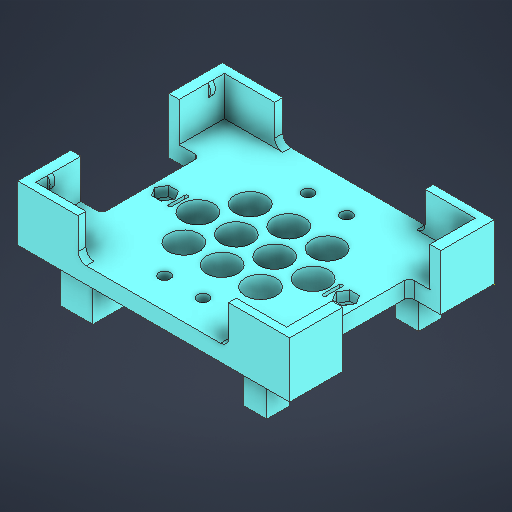
# Autodesk Inventor part: PILLARSCELLCASE18650
Saved by Autodesk Inventor 2026.2 (Build 302298000, 298)
## iProperties
Created: 2024-11-21
Part Number: PILLARSCELLCASE18650
Material: Generic
Document SubType Name: Modeling
Designer: cbast
Density: 1 g/cm^3
Appearance: Default
Mass: 190.937 g
Surface Area: 666.623 cm^2
Volume: 190.937 cm^3
Author: cbast
## iProperties of the stored document BatteryCasev1_3DPrint.ipt
Created: 2025-01-30
Part Number: BatteryCasev1_3DPrint
Material: Generic
Document SubType Name: Modeling
Designer: cbast
Density: 1 g/cm^3
Appearance: Default
Author: cbast
Autodesk Inventor part; units mm, degrees
ref_plane "YZ Plane" through (0, 0, 0) normal (1, 0, 0) x (0, 1, 0)
ref_plane "XZ Plane" through (0, 0, 0) normal (0, 1, 0) x (-1, 0, 0)
ref_plane "XY Plane" through (0, 0, 0) normal (0, 0, 1) x (1, 0, 0)
sketch "Sketch1" plane through (0, 0, 0) normal (0, 1, 0) x (-1, 0, 0)
  circle A0 centre (0, 0) radius 9.5
  circle A1 centre (23.5, 0) radius 9.5
  circle A2 centre (-23.5, 0) radius 9.5
  circle A3 centre (47, 0) radius 9.5
  line L0 (0, 0) -> (-32.9562, 0) construction
  line L1 (-32.9562, 0) -> (61.076, 0) construction
  circle A4 centre (0, 0) radius 14 construction
  circle A5 centre (-23.5, 0) radius 14 construction
  circle A6 centre (47, 0) radius 14 construction
  circle A7 centre (23.5, 0) radius 14 construction
  circle A8 centre (47, 0) radius 15 construction
  circle A9 centre (-23.5, 0) radius 15 construction
  circle A10 centre (0, 0) radius 15 construction
  circle A11 centre (23.5, 0) radius 15 construction
  line L2 (37.5, 0) -> (33, 0) construction
  circle A12 centre (35.25, -20.3516) radius 9.5
  circle A13 centre (35.25, -20.3516) radius 14 construction
  circle A14 centre (35.25, -20.3516) radius 15 construction
  line L3 (14, 0) -> (9.5, 0) construction
  line L4 (-9.5, 0) -> (-14, 0) construction
  line L5 (35.25, -20.3516) -> (-11.75, -20.3516) construction
  circle A15 centre (11.75, -20.3516) radius 9.5
  circle A16 centre (-11.75, -20.3516) radius 9.5
  circle A17 centre (11.75, -20.3516) radius 14 construction
  circle A18 centre (11.75, -20.3516) radius 15 construction
  circle A19 centre (-11.75, -20.3516) radius 14 construction
  circle A20 centre (-11.75, -20.3516) radius 15 construction
  circle A21 centre (35.25, 20.3516) radius 9.5
  circle A22 centre (35.25, 20.3516) radius 14 construction
  circle A23 centre (35.25, 20.3516) radius 15 construction
  line L6 (35.25, 20.3516) -> (-11.75, 20.3516) construction
  circle A24 centre (11.75, 20.3516) radius 9.5
  circle A25 centre (-11.75, 20.3516) radius 9.5
  circle A26 centre (11.75, 20.3516) radius 14 construction
  circle A27 centre (11.75, 20.3516) radius 15 construction
  circle A28 centre (-11.75, 20.3516) radius 14 construction
  circle A29 centre (-11.75, 20.3516) radius 15 construction
  arc A30 (49.1998, -14.8378) -> (49.1998, 14.8378) centre (47, 0) ccw
  arc A31 (49.1998, 14.8378) -> (23.5, 29.6756) centre (35.25, 20.3516) ccw
  arc A32 (23.5, 29.6756) -> (0, 29.6756) centre (11.75, 20.3516) ccw
  arc A33 (0, 29.6756) -> (-25.6998, 14.8378) centre (-11.75, 20.3516) ccw
  arc A34 (-25.6998, 14.8378) -> (-25.6998, -14.8378) centre (-23.5, 0) ccw
  arc A35 (-25.6998, -14.8378) -> (0, -29.6756) centre (-11.75, -20.3516) ccw
  arc A36 (0, -29.6756) -> (23.5, -29.6756) centre (11.75, -20.3516) ccw
  arc A37 (23.5, -29.6756) -> (49.1998, -14.8378) centre (35.25, -20.3516) ccw
  point P0 (46.8931, -14.9996)
  point P1 (46.8931, 14.9996)
  point P2 (-23.3931, 14.9996)
  point P3 (-23.3931, -14.9996)
  dimension "d145" = 28
  dimension "d149" = 28
  dimension "d0" = 19
  dimension "d2" = 19
  dimension "d4" = 19
  dimension "d53" = 19
  dimension "d144" = 28
  dimension "d150" = 28
  dimension "d154" = 30
  dimension "d158" = 30
  dimension "d162" = 30
  dimension "d163" = 30
  dimension "d291" = 19
  dimension "d292" = 28
  dimension "d293" = 30
  dimension "d294" = 19
  dimension "d295" = 19
  dimension "d296" = 28
  dimension "d297" = 30
  dimension "d298" = 28
  dimension "d299" = 30
  constraints: 40 point on circle, 36 centre point, 32 coincident, 12 end point, 10 vertical alignment, 9 equal radius, 4 tangent, 2 horizontal alignment, 1 horizontal, 1 midpoint, 1 parallel, 1 point on line, 17 other
  measures "d0" diameter of A0
  measures "d2" diameter of A1
  measures "d4" diameter of A2
  measures "d53" diameter of A3
  measures "d144" diameter of A4
  measures "d150" diameter of A7
  measures "d154" diameter of A8
  measures "d158" diameter of A9
  measures "d162" diameter of A10
  measures "d163" diameter of A11
  measures "d291" diameter of A12
  measures "d292" diameter of A13
  measures "d293" diameter of A14
  measures "d294" diameter of A15
  measures "d295" diameter of A16
  measures "d296" diameter of A17
  measures "d297" diameter of A18
  measures "d298" diameter of A19
  measures "d299" diameter of A20
extrude "Extrusion1" add sketch "Sketch1" along normal blind 15
sketch "Sketch26" plane through (0, 15, 0) normal (0, 1, 0) x (1, 0, 0)
  arc A0 (-49.1998, -14.8378) -> (-23.5, -29.6756) centre (-35.25, -20.3516) ccw projected
  arc A1 (-23.5, -29.6756) -> (0, -29.6756) centre (-11.75, -20.3516) ccw projected
  arc A2 (0, -29.6756) -> (25.6998, -14.8378) centre (11.75, -20.3516) ccw projected
  arc A3 (25.6998, -14.8378) -> (25.6998, 14.8378) centre (23.5, 0) ccw projected
  arc A4 (25.6998, 14.8378) -> (0, 29.6756) centre (11.75, 20.3516) ccw projected
  arc A5 (0, 29.6756) -> (-23.5, 29.6756) centre (-11.75, 20.3516) ccw projected
  arc A6 (-23.5, 29.6756) -> (-49.1998, 14.8378) centre (-35.25, 20.3516) ccw projected
  arc A7 (-49.1998, 14.8378) -> (-49.1998, -14.8378) centre (-47, 0) ccw projected
  circle A8 centre (0, 0) radius 9.5 projected
  circle A9 centre (-23.5, 0) radius 9.5 projected
  circle A10 centre (11.75, -20.3516) radius 9.5 projected
  circle A11 centre (-11.75, -20.3516) radius 9.5 projected
  circle A12 centre (-35.25, -20.3516) radius 9.5 projected
  circle A13 centre (11.75, 20.3516) radius 9.5 projected
  circle A14 centre (-11.75, 20.3516) radius 9.5 projected
  circle A15 centre (-35.25, 20.3516) radius 9.5 projected
  circle A16 centre (-47, 0) radius 9.5 projected
  circle A17 centre (23.5, 0) radius 9.5 projected
  line L0 (-88.45, 57.7) -> (64.95, 57.7)
  line L1 (64.95, 57.7) -> (64.95, -57.7)
  line L2 (64.95, -57.7) -> (-88.45, -57.7)
  line L3 (-88.45, -57.7) -> (-88.45, 57.7)
  line L4 (-88.45, 57.7) -> (64.95, -57.7) construction
  line L5 (64.95, 57.7) -> (-88.45, -57.7) construction
  line L6 (-88.45, 0) -> (-62, 0) construction
  line L7 (38.5, 0) -> (64.95, 0) construction
  point P0 (-11.75, 0)
  dimension "d300" = 153.4
  dimension "d301" = 115.4
  constraints: 16 end point, 4 midpoint, 3 equal length, 2 horizontal, 2 point on circle, 1 collinear, 1 perpendicular
  measures "d300" distance of L1.end L2.end
  measures "d301" distance of L0.end L1.end
extrude "Extrusion24" add sketch "Sketch26" against normal blind 10 contours L0 L1 L2 L3
sketch "Sketch28" plane through (0, 15, 0) normal (0, 1, 0) x (1, 0, 0)
  line L0 (-88.45, -57.7) -> (64.95, -57.7) projected
  line L1 (64.95, -57.7) -> (64.95, 57.7) projected
  line L2 (64.95, 57.7) -> (-88.45, 57.7) projected
  line L3 (-88.45, 57.7) -> (-88.45, -57.7) projected
  circle A0 centre (0, 0) radius 9.5 projected
  circle A1 centre (-23.5, 0) radius 9.5 projected
  circle A2 centre (11.75, -20.3516) radius 9.5 projected
  circle A3 centre (-11.75, -20.3516) radius 9.5 projected
  circle A4 centre (-35.25, -20.3516) radius 9.5 projected
  circle A5 centre (11.75, 20.3516) radius 9.5 projected
  circle A6 centre (-11.75, 20.3516) radius 9.5 projected
  circle A7 centre (-35.25, 20.3516) radius 9.5 projected
  circle A8 centre (-47, 0) radius 9.5 projected
  circle A9 centre (23.5, 0) radius 9.5 projected
  line L4 (64.95, 57.7) -> (64.95, -57.7) projected
  line L5 (-88.0641, -57.4308) -> (64.95, -57.4308)
  line L6 (64.95, -57.4308) -> (64.95, 57.7)
  line L7 (64.95, 57.7) -> (-88.0641, 57.7)
  line L8 (-88.0641, 57.7) -> (-88.0641, -57.4308)
  line L9 (-88.0641, -57.4308) -> (64.95, 57.7) construction
  line L10 (64.95, -57.4308) -> (-88.0641, 57.7) construction
  line L11 (-94.7093, -62.4308) -> (71.5952, -62.4308)
  line L12 (71.5952, -62.4308) -> (71.5952, 62.7)
  line L13 (71.5952, 62.7) -> (-94.7093, 62.7)
  line L14 (-94.7093, 62.7) -> (-94.7093, -62.4308)
  line L15 (-94.7093, -62.4308) -> (71.5952, 62.7) construction
  line L16 (71.5952, -62.4308) -> (-94.7093, 62.7) construction
  point P0 (-11.5571, 0.1346)
  point P1 (-11.5571, 0.1346)
  dimension "d306" = 5
  constraints: 24 end point, 5 midpoint, 4 parallel, 2 horizontal, 2 perpendicular, 1 point on line
  measures "d306" distance between parallel lines of L13 L2
extrude "Extrusion25" add sketch "Sketch28" along normal blind 24 and the other way blind 10 contours L14 L13 L12 L11
sketch "Sketch29" plane through (-94.7093, 39, 62.4308) normal (0, 0, 1) x (1, 0, 0)
  line L0 (6.2593, -24) -> (159.6593, -24) projected
  line L1 (41.9593, -24) -> (123.9593, -24)
  line L2 (166.3046, 0) -> (0, 0) projected
  line L3 (128.9593, -24) -> (36.9593, -24)
  line L4 (36.9593, -19) -> (36.9593, 0)
  line L5 (36.9593, 0) -> (128.9593, 0)
  line L6 (128.9593, 0) -> (128.9593, -19)
  arc A0 (36.9593, -19) -> (41.9593, -24) centre (41.9593, -19) ccw
  arc A1 (123.9593, -24) -> (128.9593, -19) centre (123.9593, -19) ccw
  point P0 (94.7093, -39)
  point P1 (82.9593, -24)
  point P2 (42.9593, -24)
  point P3 (128.9593, 0)
  dimension "d311" = 86
  dimension "d312" = 5
  constraints: 10 end point, 6 point on line, 4 point on circle, 4 tangent, 2 centre point, 2 midpoint, 2 parallel, 1 equal radius, 1 horizontal, 1 perpendicular
  measures "d311" distance of point (42.959, -24) L3.start
  measures "d312" radius of A0
extrude "Extrusion26" cut sketch "Sketch29" against normal through all
sketch "Sketch30" plane through (0, 39, 0) normal (0, 1, 0) x (1, 0, 0)
  circle A0 centre (-47, 0) radius 9.5 projected
  circle A1 centre (0, 0) radius 9.5 projected
  circle A2 centre (-23.5, 0) radius 9.5 projected
  circle A3 centre (11.75, -20.3516) radius 9.5 projected
  circle A4 centre (-11.75, -20.3516) radius 9.5 projected
  circle A5 centre (-35.25, -20.3516) radius 9.5 projected
  circle A6 centre (11.75, 20.3516) radius 9.5 projected
  circle A7 centre (-11.75, 20.3516) radius 9.5 projected
  circle A8 centre (-35.25, 20.3516) radius 9.5 projected
  circle A9 centre (23.5, 0) radius 9.5 projected
  line L0 (29.25, -57.7) -> (64.95, -57.7) projected
  line L1 (64.95, -57.7) -> (64.95, 57.7) projected
  line L2 (64.95, 57.7) -> (29.25, 57.7) projected
  line L3 (29.25, 57.7) -> (29.25, 62.7) projected
  line L4 (-52.75, 62.7) -> (29.25, 62.7) projected
  line L5 (-52.75, 57.7) -> (-52.75, 62.7) projected
  line L6 (-52.75, 57.7) -> (-88.45, 57.7) projected
  line L7 (-88.45, 57.7) -> (-88.45, -57.7) projected
  line L8 (-88.45, -57.7) -> (-52.75, -57.7) projected
  line L9 (-52.75, -62.4308) -> (-52.75, -57.7) projected
  line L10 (29.25, -62.4308) -> (-52.75, -62.4308) projected
  line L11 (29.25, -62.4308) -> (29.25, -57.7) projected
  line L12 (34.25, -57.7) -> (34.25, -62.4308) projected
  line L13 (34.25, -62.4308) -> (71.5952, -62.4308) projected
  line L14 (71.5952, -62.4308) -> (71.5952, 62.7) projected
  line L15 (71.5952, 62.7) -> (34.25, 62.7) projected
  line L16 (34.25, 62.7) -> (34.25, 57.7) projected
  line L17 (34.25, 57.7) -> (64.95, 57.7) projected
  line L18 (64.95, 57.7) -> (64.95, -57.7) projected
  line L19 (64.95, -57.7) -> (34.25, -57.7) projected
  line L20 (-88.45, -57.7) -> (-88.45, 57.7) projected
  line L21 (-57.75, -62.4308) -> (-57.75, -57.7) projected
  line L22 (-57.75, -57.7) -> (-88.45, -57.7) projected
  line L23 (-88.45, -57.7) -> (-88.45, 57.7) projected
  line L24 (-88.45, 57.7) -> (-57.75, 57.7) projected
  line L25 (-57.75, 57.7) -> (-57.75, 62.7) projected
  line L26 (-57.75, 62.7) -> (-94.7093, 62.7) projected
  line L27 (-94.7093, 62.7) -> (-94.7093, -62.4308) projected
  line L28 (-94.7093, -62.4308) -> (-57.75, -62.4308) projected
  line L29 (-88.45, -30) -> (-88.45, 30)
  line L30 (-94.7093, -62.4308) -> (-94.7093, 62.7) projected
  line L31 (-75.7093, 27) -> (-75.7093, -27)
  arc A10 (-75.7093, 27) -> (-78.7093, 30) centre (-78.7093, 27) ccw
  arc A11 (-78.7093, -30) -> (-75.7093, -27) centre (-78.7093, -27) ccw
  line L32 (-94.7093, 0) -> (-47, 0) construction
  line L33 (-47, 0) -> (-94.7093, 0) construction
  line L34 (-78.7093, 30) -> (-114.521, 30)
  line L35 (-114.521, 30) -> (-114.521, -30)
  line L36 (-114.521, -30) -> (-78.7093, -30)
  point P0 (-88.45, 0)
  dimension "d317" = 3
  constraints: 14 end point, 4 point on circle, 3 perpendicular, 2 centre point, 2 midpoint, 2 tangent, 1 collinear, 1 equal radius, 1 horizontal
  measures "d317" radius of A10
extrude "Extrusion27" cut sketch "Sketch30" against normal through all contours L36 L27 L34 L7 | L7 L34 A10 L31 A11 L36 | L36 L35 L34 L27
ref_plane "Work Plane9" through (-11.75, 15, -57.7) normal (-1, 0, 0) x (0, 0, 1)
sketch "Sketch31" plane through (0, 15, 0) normal (0, 1, 0) x (1, 0, 0)
  line L0 (-64.06, 5.3) -> (-61, 0)
  line L1 (-61, 0) -> (-64.06, -5.3)
  line L2 (-64.06, -5.3) -> (-70.1799, -5.3)
  line L3 (-70.1799, -5.3) -> (-73.2398, 0)
  line L4 (-73.2398, 0) -> (-70.1799, 5.3)
  line L5 (-70.1799, 5.3) -> (-64.06, 5.3)
  line L6 (-88.45, 57.7) -> (-57.75, 57.7) projected
  circle A0 centre (-47, 0) radius 9.5 projected
  line L7 (-57.75, -57.7) -> (-88.45, -57.7) projected
  line L8 (-75.7093, -27) -> (-75.7093, 27) construction
  line L9 (-75.7093, 0) -> (-47, 0) construction
  point P0 (0, 0)
  point P1 (-67.1199, 0)
  dimension "d323" = 14
  dimension "d332" = 10.6
  constraints: 14 end point, 2 parallel, 1 midpoint, 1 perpendicular, 1 point on line, 13 other
  measures "d323" distance of L9.end L0.end
  measures "d332" distance between parallel lines of L2 L5
extrude "Extrusion28" cut sketch "Sketch31" against normal blind 6 contours L0 L1 L2 L3 L4 L5
sketch "Sketch32" plane through (0, 9, 0) normal (0, 1, 0) x (1, 0, 0)
  line L0 (-73.2398, 0) -> (-70.1799, 5.3) projected
  line L1 (-70.1799, -5.3) -> (-73.2398, 0) projected
  line L2 (-64.06, -5.3) -> (-70.1799, -5.3) projected
  line L3 (-61, 0) -> (-64.06, -5.3) projected
  line L4 (-64.06, 5.3) -> (-61, 0) projected
  line L5 (-70.1799, 5.3) -> (-64.06, 5.3) projected
  circle A0 centre (-67.1199, 0) radius 3.25
  line L6 (-63.8699, 0) -> (-61, 0) construction
  line L7 (-70.3699, 0) -> (-73.2398, 0) construction
  point P0 (0, 0)
  dimension "d329" = 6.5
  constraints: 4 end point, 2 collinear, 2 point on circle, 1 centre point, 1 horizontal, 1 point on line
  measures "d329" diameter of A0
extrude "Extrusion29" cut sketch "Sketch32" against normal through all contours A0
sketch "Sketch33" plane through (0, 15, 0) normal (0, 1, 0) x (1, 0, 0)
  line L0 (-70.1799, -5.3) -> (-73.2398, 0) projected
  line L1 (-73.2398, 0) -> (-70.1799, 5.3) projected
  line L2 (-70.1799, 5.3) -> (-64.06, 5.3) projected
  line L3 (-64.06, 5.3) -> (-61, 0) projected
  line L4 (-61, 0) -> (-64.06, -5.3) projected
  line L5 (-64.06, -5.3) -> (-70.1799, -5.3) projected
  circle A0 centre (23.5, 0) radius 9.5 projected
  circle A1 centre (-35.25, 20.3516) radius 9.5 projected
  circle A2 centre (-11.75, 20.3516) radius 9.5 projected
  circle A3 centre (11.75, 20.3516) radius 9.5 projected
  circle A4 centre (-35.25, -20.3516) radius 9.5 projected
  circle A5 centre (-11.75, -20.3516) radius 9.5 projected
  circle A6 centre (11.75, -20.3516) radius 9.5 projected
  circle A7 centre (-23.5, 0) radius 9.5 projected
  circle A8 centre (0, 0) radius 9.5 projected
  circle A9 centre (-47, 0) radius 9.5 projected
  line L6 (64.95, -57.7) -> (64.95, 57.7) projected
  line L7 (64.95, 57.7) -> (29.25, 57.7) projected
  line L8 (29.25, 57.7) -> (29.25, 62.7) projected
  line L9 (-52.75, 62.7) -> (29.25, 62.7) projected
  line L10 (-52.75, 57.7) -> (-52.75, 62.7) projected
  line L11 (-52.75, 57.7) -> (-88.45, 57.7) projected
  line L12 (-88.45, 57.7) -> (-88.45, 30) projected
  line L13 (-88.45, -57.7) -> (-52.75, -57.7) projected
  line L14 (-52.75, -62.4308) -> (-52.75, -57.7) projected
  line L15 (29.25, -62.4308) -> (-52.75, -62.4308) projected
  line L16 (29.25, -62.4308) -> (29.25, -57.7) projected
  line L17 (29.25, -57.7) -> (64.95, -57.7) projected
  line L18 (-59, 6) -> (-59, -6) construction
  line L19 (-60, 5) -> (-60, -5)
  line L20 (-58, -5) -> (-58, 5)
  arc A10 (-58, 5) -> (-60, 5) centre (-59, 5) ccw
  arc A11 (-60, -5) -> (-58, -5) centre (-59, -5) ccw
  line L21 (-47, 0) -> (-75.7093, 0) construction
  line L22 (-88.45, 30) -> (-78.7093, 30) projected
  arc A12 (-75.7093, 27) -> (-78.7093, 30) centre (-78.7093, 27) ccw projected
  line L23 (-75.7093, 27) -> (-75.7093, -27) projected
  arc A13 (-78.7093, -30) -> (-75.7093, -27) centre (-78.7093, -27) ccw projected
  line L24 (-78.7093, -30) -> (-88.45, -30) projected
  line L25 (-88.45, -30) -> (-88.45, -57.7) projected
  point P0 (-59, 0)
  dimension "d333" = 12
  dimension "d334" = 2
  dimension "d335" = 11
  constraints: 10 end point, 6 point on circle, 4 tangent, 3 point on line, 2 centre point, 1 midpoint, 1 parallel, 1 vertical
  measures "d333" distance of L18.start L18.end
  measures "d334" diameter of A11
  measures "d335" distance from line of L20 L21.start
extrude "Extrusion30" cut sketch "Sketch33" against normal through all contours A10 L20 A11 L19
mirror "Mirror9" about plane through (-11.75, 15, -57.7) normal (-1, 0, 0) of "Extrusion28", "Extrusion29", "Extrusion30"
ref_plane "Work Plane10" through (-94.7093, 5, -0.1346) normal (0, 0, 1) x (1, 0, 0)
ref_plane "Work Plane11" through (64.95, 15, -47.7) normal (0, 0, 1) x (1, 0, 0)
sketch "Sketch34" plane through (64.95, 15, -47.7) normal (0, 0, 1) x (1, 0, 0)
  line L0 (0, 24) -> (0, 0) projected
  line L1 (0, 0) -> (0, 16) construction
  line L2 (0, 0) -> (0, 24) construction
  line L3 (0, 16) -> (0, 24)
  arc A0 (0, 24) -> (0, 16) centre (0, 20) ccw
  arc A1 (0, 24) -> (0, 16) centre (4.4721, 20) ccw
  point P0 (-64.95, -15)
  dimension "d339" = 16
  dimension "d340" = 8
  dimension "d342" = 6
  constraints: 4 end point, 4 point on circle, 2 centre point, 2 point on line
  measures "d339" distance of L0.end L1.end
  measures "d340" distance of L1.end L3.end
  measures "d342" radius of A1
extrude "Extrusion31" add sketch "Sketch34" against normal blind 3 contours L0 A1
mirror "Mirror10" about plane through (-11.75, 15, -57.7) normal (-1, 0, 0) of "Extrusion31"
mirror "Mirror11" about plane through (-94.7093, 5, -0.1346) normal (0, 0, 1) of "Extrusion31", "Mirror10"
sketch "Sketch35" plane through (0, 5, 0) normal (0, -1, 0) x (1, 0, 0)
  line L0 (-94.7093, -62.7) -> (71.5952, -62.7) projected
  point P0 (0, 0)
sketch "Sketch36" plane through (0, 15, 0) normal (0, 1, 0) x (1, 0, 0)
  line L0 (-88.45, 30) -> (-78.7093, 30) construction
  line L1 (-78.7093, -30) -> (-88.45, -30) construction
  line L2 (-75.7093, 27) -> (-75.7093, -27) construction
  line L3 (64.95, 47.7) -> (64.95, -47.4308) construction
  line L4 (71.5952, 62.7) -> (71.5952, -62.4308) construction
  line L5 (64.95, 20.5623) -> (52.209, 20.5623) construction
  line L6 (-75.7093, -2.0148) -> (-75.7093, -47.4308) construction
  line L7 (52.24, 27) -> (52.24, -27)
  line L8 (55.24, -30) -> (114.3089, -30)
  line L9 (114.3089, -30) -> (114.3089, 30)
  line L10 (114.3089, 30) -> (55.24, 30)
  arc A0 (55.24, 30) -> (52.24, 27) centre (55.24, 27) ccw
  arc A1 (52.24, -27) -> (55.24, -30) centre (55.24, -27) ccw
  point P0 (0, 0)
  dimension "d347" = 12.741
  dimension "d348" = 3
  constraints: 12 end point, 4 point on circle, 4 tangent, 3 perpendicular, 3 point on line, 2 centre point, 1 equal radius, 1 horizontal, 1 vertical
  measures "d347" distance of L5.start L5.end
  measures "d348" radius of A0
extrude "Extrusion32" cut sketch "Sketch36" along normal through all both and the other way through all
sketch "Sketch37" plane through (0, 5, 0) normal (0, -1, 0) x (1, 0, 0)
  line L0 (-72.2093, 38.9308) -> (-57.2093, 38.9308)
  line L1 (-57.2093, 38.9308) -> (-57.2093, 53.9308)
  line L2 (-57.2093, 53.9308) -> (-72.2093, 53.9308)
  line L3 (-72.2093, 53.9308) -> (-72.2093, 38.9308)
  line L4 (-72.2093, 38.9308) -> (-57.2093, 53.9308) construction
  line L5 (-57.2093, 38.9308) -> (-72.2093, 53.9308) construction
  line L6 (-74.7093, 36.4308) -> (-54.7093, 36.4308)
  line L7 (-54.7093, 36.4308) -> (-54.7093, 56.4308)
  line L8 (-54.7093, 56.4308) -> (-74.7093, 56.4308)
  line L9 (-74.7093, 56.4308) -> (-74.7093, 36.4308)
  line L10 (-74.7093, 36.4308) -> (-54.7093, 56.4308) construction
  line L11 (-54.7093, 36.4308) -> (-74.7093, 56.4308) construction
  line L12 (-94.7093, 62.4308) -> (-94.7093, 30) projected
  line L13 (71.5952, 62.4308) -> (-94.7093, 62.4308) projected
  line L14 (34.5952, 39.4308) -> (48.5952, 39.4308)
  line L15 (48.5952, 39.4308) -> (48.5952, 53.4308)
  line L16 (48.5952, 53.4308) -> (34.5952, 53.4308)
  line L17 (34.5952, 53.4308) -> (34.5952, 39.4308)
  line L18 (34.5952, 39.4308) -> (48.5952, 53.4308) construction
  line L19 (48.5952, 39.4308) -> (34.5952, 53.4308) construction
  line L20 (71.5952, 30) -> (71.5952, 62.4308) projected
  line L21 (-75.7093, -27) -> (-75.7093, 27) construction
  line L22 (-75.7093, 0) -> (52.24, 0) construction
  line L23 (52.24, -27) -> (52.24, 27) construction
  line L24 (-72.2093, -38.9308) -> (-57.2093, -38.9308)
  line L25 (-57.2093, -38.9308) -> (-57.2093, -53.9308)
  line L26 (-57.2093, -53.9308) -> (-72.2093, -53.9308)
  line L27 (-72.2093, -53.9308) -> (-72.2093, -38.9308)
  line L28 (-72.2093, -38.9308) -> (-57.2093, -53.9308) construction
  line L29 (-57.2093, -38.9308) -> (-72.2093, -53.9308) construction
  line L30 (-74.7093, -36.4308) -> (-54.7093, -36.4308)
  line L31 (-54.7093, -36.4308) -> (-54.7093, -56.4308)
  line L32 (-54.7093, -56.4308) -> (-74.7093, -56.4308)
  line L33 (-74.7093, -56.4308) -> (-74.7093, -36.4308)
  line L34 (-74.7093, -36.4308) -> (-54.7093, -56.4308) construction
  line L35 (-54.7093, -36.4308) -> (-74.7093, -56.4308) construction
  line L36 (34.5952, -39.4308) -> (48.5952, -39.4308)
  line L37 (48.5952, -39.4308) -> (48.5952, -53.4308)
  line L38 (48.5952, -53.4308) -> (34.5952, -53.4308)
  line L39 (34.5952, -53.4308) -> (34.5952, -39.4308)
  line L40 (34.5952, -39.4308) -> (48.5952, -53.4308) construction
  line L41 (48.5952, -39.4308) -> (34.5952, -53.4308) construction
  point P0 (0, 0)
  point P1 (-64.7093, 46.4308)
  point P2 (41.5952, 46.4308)
  point P3 (-64.7093, -46.4308)
  point P4 (41.5952, -46.4308)
  dimension "d351" = 15
  dimension "d352" = 20
  dimension "d355" = 16
  dimension "d356" = 30
  dimension "d357" = 14
  dimension "d358" = 14
  dimension "d359" = 16
  dimension "d360" = 30
  constraints: 74 end point, 14 symmetric about line, 8 midpoint, 6 parallel, 4 perpendicular, 3 horizontal, 2 point on line
  measures "d351" distance of L2.end L0.start
  measures "d352" distance of L8.end L6.start
  measures "d355" distance from line of L13 point (-64.709, 46.431)
  measures "d356" distance from line of point (-64.709, 46.431) L12
  measures "d357" distance of L15.end L16.end
  measures "d358" distance of L16.end L14.start
  measures "d359" distance from line of point (41.595, 46.431) L13
  measures "d360" distance from line of L20 point (41.595, 46.431)
extrude "Extrusion33" add sketch "Sketch37" along normal blind 25
sketch "Sketch38" plane through (0, 5, 0) normal (0, -1, 0) x (1, 0, 0)
  line L0 (-72.2093, 38.9308) -> (-57.2093, 38.9308) projected
  line L1 (-57.2093, 38.9308) -> (-57.2093, 53.9308) projected
  line L2 (-57.2093, 53.9308) -> (-72.2093, 53.9308) projected
  line L3 (-72.2093, 53.9308) -> (-72.2093, 38.9308) projected
  line L4 (-57.2093, -53.9308) -> (-57.2093, -38.9308) projected
  line L5 (-57.2093, -38.9308) -> (-72.2093, -38.9308) projected
  line L6 (-72.2093, -38.9308) -> (-72.2093, -53.9308) projected
  line L7 (-72.2093, -53.9308) -> (-57.2093, -53.9308) projected
  line L8 (-72.2093, 53.9308) -> (-57.2093, 53.9308)
  line L9 (-57.2093, 53.9308) -> (-57.2093, 38.9308)
  line L10 (-57.2093, 38.9308) -> (-72.2093, 38.9308)
  line L11 (-72.2093, 38.9308) -> (-72.2093, 53.9308)
  line L12 (-72.2093, -38.9308) -> (-57.2093, -38.9308)
  line L13 (-57.2093, -38.9308) -> (-57.2093, -53.9308)
  line L14 (-57.2093, -53.9308) -> (-72.2093, -53.9308)
  line L15 (-72.2093, -53.9308) -> (-72.2093, -38.9308)
  point P0 (0, 0)
  constraints: 16 end point, 4 parallel, 2 horizontal, 2 perpendicular
extrude "Extrusion34" add sketch "Sketch38" along normal blind 12.5
sketch "Sketch39" plane through (0, 5, 0) normal (0, -1, 0) x (1, 0, 0)
  line L0 (-23.519, 60.7587) -> (0.6762, 60.7587) construction
  line L1 (0.6762, 60.7587) -> (0.6762, 41.0836) construction
  line L2 (0.6762, 41.0836) -> (-23.519, 41.0836) construction
  line L3 (-23.519, 41.0836) -> (-23.519, 60.7587) construction
  line L4 (-21.6935, 57.6543) -> (-20.6628, 60.7043)
  line L5 (-20.6628, 60.7043) -> (-19.8274, 60.7043)
  line L6 (-19.8274, 60.7043) -> (-18.7967, 57.6543)
  line L7 (-18.7967, 57.6543) -> (-19.5852, 57.6543)
  line L8 (-19.5852, 57.6543) -> (-19.7755, 58.2772)
  line L9 (-19.7755, 58.2772) -> (-20.7345, 58.2772)
  line L10 (-20.7345, 58.2772) -> (-20.9273, 57.6543)
  line L11 (-20.9273, 57.6543) -> (-21.6935, 57.6543)
  line L12 (-19.9436, 58.8308) -> (-20.255, 59.8393)
  line L13 (-20.255, 59.8393) -> (-20.5689, 58.8308)
  line L14 (-20.5689, 58.8308) -> (-19.9436, 58.8308)
  line L15 (-15.6751, 57.6543) -> (-16.6069, 57.6543)
  line L16 (-16.6069, 57.6543) -> (-17.4546, 58.774)
  line L17 (-17.4546, 58.774) -> (-17.7315, 58.774)
  line L18 (-17.7315, 58.774) -> (-17.7315, 57.6543)
  line L19 (-17.7315, 57.6543) -> (-18.4927, 57.6543)
  line L20 (-18.4927, 57.6543) -> (-18.4927, 60.7043)
  line L21 (-18.4927, 60.7043) -> (-17.2668, 60.7043)
  spline S0 degree 2 poles (-17.2668, 60.7043) (-17.0122, 60.7043) (-16.6365, 60.6401) (-16.4759, 60.5412) knots 0 0 0 1 2 2 2
  spline S1 degree 2 poles (-16.4759, 60.5412) (-16.3127, 60.4374) (-16.12, 60.1136) (-16.12, 59.8665) knots 0 0 0 1 2 2 2
  spline S2 degree 2 poles (-16.12, 59.8665) (-16.12, 59.518) (-16.4363, 59.0805) (-16.7008, 58.952) knots 0 0 0 1 2 2 2
  line L22 (-16.7008, 58.952) -> (-15.6751, 57.6543)
  spline S3 degree 2 poles (-16.9059, 59.7701) (-16.9059, 59.8862) (-16.9949, 60.0518) (-17.0963, 60.0963) knots 0 0 0 1 2 2 2
  spline S4 degree 2 poles (-17.0963, 60.0963) (-17.1679, 60.126) (-17.3434, 60.1433) (-17.4744, 60.1433) knots 0 0 0 1 2 2 2
  line L23 (-17.4744, 60.1433) -> (-17.7315, 60.1433)
  line L24 (-17.7315, 60.1433) -> (-17.7315, 59.3227)
  line L25 (-17.7315, 59.3227) -> (-17.5115, 59.3227)
  spline S5 degree 2 poles (-17.5115, 59.3227) (-17.3533, 59.3227) (-17.1284, 59.3622) (-17.0518, 59.424) knots 0 0 0 1 2 2 2
  spline S6 degree 2 poles (-17.0518, 59.424) (-16.9776, 59.4834) (-16.9059, 59.6415) (-16.9059, 59.7701) knots 0 0 0 1 2 2 2
  line L26 (-14.8619, 57.6543) -> (-14.8619, 60.1235)
  line L27 (-14.8619, 60.1235) -> (-15.764, 60.1235)
  line L28 (-15.764, 60.1235) -> (-15.764, 60.7043)
  line L29 (-15.764, 60.7043) -> (-13.1935, 60.7043)
  line L30 (-13.1935, 60.7043) -> (-13.1935, 60.1235)
  line L31 (-13.1935, 60.1235) -> (-14.0957, 60.1235)
  line L32 (-14.0957, 60.1235) -> (-14.0957, 57.6543)
  line L33 (-14.0957, 57.6543) -> (-14.8619, 57.6543)
  spline S7 degree 2 poles (-11.938, 57.6) (-12.2889, 57.6) (-12.8179, 57.7359) (-13.0452, 57.8348) knots 0 0 0 1 2 2 2
  line L34 (-13.0452, 57.8348) -> (-13.0452, 58.5614)
  line L35 (-13.0452, 58.5614) -> (-12.976, 58.5614)
  spline S8 degree 2 poles (-12.976, 58.5614) (-12.7462, 58.3662) (-12.195, 58.1561) (-11.9355, 58.1561) knots 0 0 0 1 2 2 2
  spline S9 degree 2 poles (-11.9355, 58.1561) (-11.8687, 58.1561) (-11.6537, 58.1857) (-11.5894, 58.2154) knots 0 0 0 1 2 2 2
  spline S10 degree 2 poles (-11.5894, 58.2154) (-11.5104, 58.25) (-11.3991, 58.3761) (-11.3991, 58.4774) knots 0 0 0 1 2 2 2
  spline S11 degree 2 poles (-11.3991, 58.4774) (-11.3991, 58.5936) (-11.5796, 58.7369) (-11.7031, 58.7691) knots 0 0 0 1 2 2 2
  spline S12 degree 2 poles (-11.7031, 58.7691) (-11.8589, 58.8111) (-12.2123, 58.8827) (-12.368, 58.9371) knots 0 0 0 1 2 2 2
  spline S13 degree 2 poles (-12.368, 58.9371) (-12.7215, 59.0607) (-13.0279, 59.4834) (-13.0279, 59.7997) knots 0 0 0 1 2 2 2
  spline S14 degree 2 poles (-13.0279, 59.7997) (-13.0279, 60.2273) (-12.3038, 60.7587) (-11.76, 60.7587) knots 0 0 0 1 2 2 2
  spline S15 degree 2 poles (-11.76, 60.7587) (-11.4881, 60.7587) (-10.9493, 60.6475) (-10.7367, 60.5536) knots 0 0 0 1 2 2 2
  line L36 (-10.7367, 60.5536) -> (-10.7367, 59.8566)
  line L37 (-10.7367, 59.8566) -> (-10.8035, 59.8566)
  spline S16 degree 2 poles (-10.8035, 59.8566) (-10.974, 60.0024) (-11.4634, 60.2026) (-11.7204, 60.2026) knots 0 0 0 1 2 2 2
  spline S17 degree 2 poles (-11.7204, 60.2026) (-11.8218, 60.2026) (-11.98, 60.1729) (-12.0689, 60.1334) knots 0 0 0 1 2 2 2
  spline S18 degree 2 poles (-12.0689, 60.1334) (-12.1406, 60.1013) (-12.2444, 59.9727) (-12.2444, 59.8936) knots 0 0 0 1 2 2 2
  spline S19 degree 2 poles (-12.2444, 59.8936) (-12.2444, 59.775) (-12.0788, 59.6391) (-11.8416, 59.5847) knots 0 0 0 1 2 2 2
  spline S20 degree 2 poles (-11.8416, 59.5847) (-11.6883, 59.5501) (-11.4041, 59.4834) (-11.2409, 59.4265) knots 0 0 0 1 2 2 2
  spline S21 degree 2 poles (-11.2409, 59.4265) (-10.9246, 59.3103) (-10.6156, 58.9248) (-10.6156, 58.6084) knots 0 0 0 1 2 2 2
  spline S22 degree 2 poles (-10.6156, 58.6084) (-10.6156, 58.1536) (-11.3299, 57.6) (-11.938, 57.6) knots 0 0 0 1 2 2 2
  line L38 (-6.9601, 57.6543) -> (-8.9942, 57.6543)
  line L39 (-8.9942, 57.6543) -> (-8.9942, 60.7043)
  line L40 (-8.9942, 60.7043) -> (-8.228, 60.7043)
  line L41 (-8.228, 60.7043) -> (-8.228, 58.2352)
  line L42 (-8.228, 58.2352) -> (-6.9601, 58.2352)
  line L43 (-6.9601, 58.2352) -> (-6.9601, 57.6543)
  line L44 (-6.923, 57.6543) -> (-5.8923, 60.7043)
  line L45 (-5.8923, 60.7043) -> (-5.0569, 60.7043)
  line L46 (-5.0569, 60.7043) -> (-4.0262, 57.6543)
  line L47 (-4.0262, 57.6543) -> (-4.8147, 57.6543)
  line L48 (-4.8147, 57.6543) -> (-5.005, 58.2772)
  line L49 (-5.005, 58.2772) -> (-5.964, 58.2772)
  line L50 (-5.964, 58.2772) -> (-6.1568, 57.6543)
  line L51 (-6.1568, 57.6543) -> (-6.923, 57.6543)
  line L52 (-5.1731, 58.8308) -> (-5.4845, 59.8393)
  line L53 (-5.4845, 59.8393) -> (-5.7984, 58.8308)
  line L54 (-5.7984, 58.8308) -> (-5.1731, 58.8308)
  spline S23 degree 2 poles (-1.2852, 58.5886) (-1.2852, 58.3612) (-1.4582, 58.0177) (-1.6016, 57.904) knots 0 0 0 1 2 2 2
  spline S24 degree 2 poles (-1.6016, 57.904) (-1.7746, 57.768) (-2.1849, 57.6543) (-2.5037, 57.6543) knots 0 0 0 1 2 2 2
  line L55 (-2.5037, 57.6543) -> (-3.7222, 57.6543)
  line L56 (-3.7222, 57.6543) -> (-3.7222, 60.7043)
  line L57 (-3.7222, 60.7043) -> (-2.6471, 60.7043)
  spline S25 degree 2 poles (-2.6471, 60.7043) (-2.3109, 60.7043) (-1.9649, 60.6524) (-1.8141, 60.5709) knots 0 0 0 1 2 2 2
  spline S26 degree 2 poles (-1.8141, 60.5709) (-1.6485, 60.4844) (-1.4879, 60.1878) (-1.4879, 59.995) knots 0 0 0 1 2 2 2
  spline S27 degree 2 poles (-1.4879, 59.995) (-1.4879, 59.7725) (-1.7103, 59.424) (-1.908, 59.3425) knots 0 0 0 1 2 2 2
  line L58 (-1.908, 59.3425) -> (-1.908, 59.3276)
  spline S28 degree 2 poles (-1.908, 59.3276) (-1.6238, 59.2683) (-1.2852, 58.9) (-1.2852, 58.5886) knots 0 0 0 1 2 2 2
  spline S29 degree 2 poles (-2.0761, 58.601) (-2.0761, 58.7443) (-2.1898, 58.905) (-2.3035, 58.947) knots 0 0 0 1 2 2 2
  spline S30 degree 2 poles (-2.3035, 58.947) (-2.3727, 58.9742) (-2.6174, 58.9791) (-2.8201, 58.9791) knots 0 0 0 1 2 2 2
  line L59 (-2.8201, 58.9791) -> (-2.961, 58.9791)
  line L60 (-2.961, 58.9791) -> (-2.961, 58.2105)
  line L61 (-2.961, 58.2105) -> (-2.9189, 58.2105)
  spline S31 degree 2 poles (-2.9189, 58.2105) (-2.6224, 58.2105) (-2.395, 58.2179) (-2.2763, 58.2698) knots 0 0 0 1 2 2 2
  spline S32 degree 2 poles (-2.2763, 58.2698) (-2.1725, 58.3167) (-2.0761, 58.4898) (-2.0761, 58.601) knots 0 0 0 1 2 2 2
  spline S33 degree 2 poles (-2.2664, 59.8442) (-2.2664, 59.9184) (-2.3431, 60.0741) (-2.4221, 60.1087) knots 0 0 0 1 2 2 2
  spline S34 degree 2 poles (-2.4221, 60.1087) (-2.4963, 60.1433) (-2.7039, 60.1482) (-2.9091, 60.1482) knots 0 0 0 1 2 2 2
  line L62 (-2.9091, 60.1482) -> (-2.961, 60.1482)
  line L63 (-2.961, 60.1482) -> (-2.961, 59.5007)
  line L64 (-2.961, 59.5007) -> (-2.8646, 59.5007)
  spline S35 degree 2 poles (-2.8646, 59.5007) (-2.6693, 59.5007) (-2.5111, 59.5081) (-2.4271, 59.5476) knots 0 0 0 1 2 2 2
  spline S36 degree 2 poles (-2.4271, 59.5476) (-2.3356, 59.5921) (-2.2664, 59.7429) (-2.2664, 59.8442) knots 0 0 0 1 2 2 2
  spline S37 degree 2 poles (-20.711, 53.6657) (-20.711, 53.426) (-20.8742, 53.0206) (-21.0348, 52.8748) knots 0 0 0 1 2 2 2
  spline S38 degree 2 poles (-21.0348, 52.8748) (-21.1955, 52.729) (-21.6354, 52.5683) (-21.9567, 52.5683) knots 0 0 0 1 2 2 2
  spline S39 degree 2 poles (-21.9567, 52.5683) (-22.2978, 52.5708) (-22.7872, 52.682) (-22.9479, 52.7537) knots 0 0 0 1 2 2 2
  line L65 (-22.9479, 52.7537) -> (-22.9479, 53.4186)
  line L66 (-22.9479, 53.4186) -> (-22.8787, 53.4186)
  spline S40 degree 2 poles (-22.8787, 53.4186) (-22.8193, 53.3864) (-22.676, 53.3024) (-22.5598, 53.2579) knots 0 0 0 1 2 2 2
  spline S41 degree 2 poles (-22.5598, 53.2579) (-22.4511, 53.2159) (-22.2261, 53.1591) (-22.0902, 53.1591) knots 0 0 0 1 2 2 2
  spline S42 degree 2 poles (-22.0902, 53.1591) (-21.9716, 53.1591) (-21.6947, 53.2184) (-21.6107, 53.2975) knots 0 0 0 1 2 2 2
  spline S43 degree 2 poles (-21.6107, 53.2975) (-21.5489, 53.3593) (-21.4797, 53.51) (-21.4797, 53.6361) knots 0 0 0 1 2 2 2
  spline S44 degree 2 poles (-21.4797, 53.6361) (-21.4797, 53.7448) (-21.5687, 53.8981) (-21.6404, 53.945) knots 0 0 0 1 2 2 2
  spline S45 degree 2 poles (-21.6404, 53.945) (-21.7442, 54.0142) (-22.0408, 54.0538) (-22.147, 54.0538) knots 0 0 0 1 2 2 2
  spline S46 degree 2 poles (-22.147, 54.0538) (-22.3151, 54.0538) (-22.634, 53.9994) (-22.7501, 53.9698) knots 0 0 0 1 2 2 2
  line L67 (-22.7501, 53.9698) -> (-22.8169, 53.9698)
  line L68 (-22.8169, 53.9698) -> (-22.8169, 55.6826)
  line L69 (-22.8169, 55.6826) -> (-20.7951, 55.6826)
  line L70 (-20.7951, 55.6826) -> (-20.7951, 55.1067)
  line L71 (-20.7951, 55.1067) -> (-22.0927, 55.1067)
  line L72 (-22.0927, 55.1067) -> (-22.0927, 54.6)
  spline S47 degree 2 poles (-22.0927, 54.6) (-22.0309, 54.605) (-21.8603, 54.6099) (-21.8134, 54.6099) knots 0 0 0 1 2 2 2
  spline S48 degree 2 poles (-21.8134, 54.6099) (-21.5934, 54.6099) (-21.2227, 54.5209) (-21.0768, 54.4295) knots 0 0 0 1 2 2 2
  spline S49 degree 2 poles (-21.0768, 54.4295) (-20.9038, 54.3158) (-20.711, 53.9376) (-20.711, 53.6657) knots 0 0 0 1 2 2 2
  line L73 (-18.4767, 55.8185) -> (-19.6902, 51.9702)
  line L74 (-19.6902, 51.9702) -> (-20.2785, 51.9702)
  line L75 (-20.2785, 51.9702) -> (-19.0674, 55.8185)
  line L76 (-19.0674, 55.8185) -> (-18.4767, 55.8185)
  line L77 (-15.5502, 52.6326) -> (-17.792, 52.6326)
  line L78 (-17.792, 52.6326) -> (-17.792, 53.1294)
  spline S50 degree 2 poles (-17.792, 53.1294) (-17.5078, 53.3568) (-17.053, 53.7572) (-16.8825, 53.9376) knots 0 0 0 1 2 2 2
  spline S51 degree 2 poles (-16.8825, 53.9376) (-16.6575, 54.1724) (-16.4573, 54.5308) (-16.4573, 54.7187) knots 0 0 0 1 2 2 2
  spline S52 degree 2 poles (-16.4573, 54.7187) (-16.4573, 54.9312) (-16.7119, 55.1586) (-16.9393, 55.1586) knots 0 0 0 1 2 2 2
  spline S53 degree 2 poles (-16.9393, 55.1586) (-17.0555, 55.1586) (-17.2631, 55.1018) (-17.3694, 55.0573) knots 0 0 0 1 2 2 2
  spline S54 degree 2 poles (-17.3694, 55.0573) (-17.4732, 55.0103) (-17.6215, 54.9114) (-17.6586, 54.8867) knots 0 0 0 1 2 2 2
  line L79 (-17.6586, 54.8867) -> (-17.7179, 54.8867)
  line L80 (-17.7179, 54.8867) -> (-17.7179, 55.5516)
  spline S55 degree 2 poles (-17.7179, 55.5516) (-17.5893, 55.6134) (-17.0406, 55.7419) (-16.7861, 55.7419) knots 0 0 0 1 2 2 2
  spline S56 degree 2 poles (-16.7861, 55.7419) (-16.2423, 55.7419) (-15.6837, 55.2575) (-15.6837, 54.82) knots 0 0 0 1 2 2 2
  spline S57 degree 2 poles (-15.6837, 54.82) (-15.6837, 54.5506) (-15.9383, 54.0315) (-16.2324, 53.7349) knots 0 0 0 1 2 2 2
  spline S58 degree 2 poles (-16.2324, 53.7349) (-16.4178, 53.552) (-16.7663, 53.2678) (-16.8429, 53.2085) knots 0 0 0 1 2 2 2
  line L81 (-16.8429, 53.2085) -> (-15.5502, 53.2085)
  line L82 (-15.5502, 53.2085) -> (-15.5502, 52.6326)
  line L83 (-12.9451, 55.077) -> (-14.2477, 52.6326)
  line L84 (-14.2477, 52.6326) -> (-15.0979, 52.6326)
  line L85 (-15.0979, 52.6326) -> (-13.7361, 55.1067)
  line L86 (-13.7361, 55.1067) -> (-15.1894, 55.1067)
  line L87 (-15.1894, 55.1067) -> (-15.1894, 55.6826)
  line L88 (-15.1894, 55.6826) -> (-12.9451, 55.6826)
  line L89 (-12.9451, 55.6826) -> (-12.9451, 55.077)
  line L90 (-10.7133, 55.8185) -> (-11.9268, 51.9702)
  line L91 (-11.9268, 51.9702) -> (-12.5151, 51.9702)
  line L92 (-12.5151, 51.9702) -> (-11.304, 55.8185)
  line L93 (-11.304, 55.8185) -> (-10.7133, 55.8185)
  line L94 (-7.7868, 52.6326) -> (-10.0286, 52.6326)
  line L95 (-10.0286, 52.6326) -> (-10.0286, 53.1294)
  spline S59 degree 2 poles (-10.0286, 53.1294) (-9.7444, 53.3568) (-9.2896, 53.7572) (-9.119, 53.9376) knots 0 0 0 1 2 2 2
  spline S60 degree 2 poles (-9.119, 53.9376) (-8.8941, 54.1724) (-8.6939, 54.5308) (-8.6939, 54.7187) knots 0 0 0 1 2 2 2
  spline S61 degree 2 poles (-8.6939, 54.7187) (-8.6939, 54.9312) (-8.9485, 55.1586) (-9.1759, 55.1586) knots 0 0 0 1 2 2 2
  spline S62 degree 2 poles (-9.1759, 55.1586) (-9.2921, 55.1586) (-9.4997, 55.1018) (-9.606, 55.0573) knots 0 0 0 1 2 2 2
  spline S63 degree 2 poles (-9.606, 55.0573) (-9.7098, 55.0103) (-9.8581, 54.9114) (-9.8951, 54.8867) knots 0 0 0 1 2 2 2
  line L96 (-9.8951, 54.8867) -> (-9.9545, 54.8867)
  line L97 (-9.9545, 54.8867) -> (-9.9545, 55.5516)
  spline S64 degree 2 poles (-9.9545, 55.5516) (-9.8259, 55.6134) (-9.2772, 55.7419) (-9.0227, 55.7419) knots 0 0 0 1 2 2 2
  spline S65 degree 2 poles (-9.0227, 55.7419) (-8.4789, 55.7419) (-7.9203, 55.2575) (-7.9203, 54.82) knots 0 0 0 1 2 2 2
  spline S66 degree 2 poles (-7.9203, 54.82) (-7.9203, 54.5506) (-8.1749, 54.0315) (-8.469, 53.7349) knots 0 0 0 1 2 2 2
  spline S67 degree 2 poles (-8.469, 53.7349) (-8.6544, 53.552) (-9.0029, 53.2678) (-9.0795, 53.2085) knots 0 0 0 1 2 2 2
  line L98 (-9.0795, 53.2085) -> (-7.7868, 53.2085)
  line L99 (-7.7868, 53.2085) -> (-7.7868, 52.6326)
  spline S68 degree 2 poles (-5.1545, 54.1576) (-5.1545, 53.7621) (-5.2806, 53.1689) (-5.4215, 52.9687) knots 0 0 0 1 2 2 2
  spline S69 degree 2 poles (-5.4215, 52.9687) (-5.5599, 52.771) (-6.0073, 52.5683) (-6.3286, 52.5683) knots 0 0 0 1 2 2 2
  spline S70 degree 2 poles (-6.3286, 52.5683) (-6.6524, 52.5683) (-7.0972, 52.771) (-7.2381, 52.9737) knots 0 0 0 1 2 2 2
  spline S71 degree 2 poles (-7.2381, 52.9737) (-7.379, 53.1739) (-7.5051, 53.7621) (-7.5051, 54.1576) knots 0 0 0 1 2 2 2
  spline S72 degree 2 poles (-7.5051, 54.1576) (-7.5051, 54.5629) (-7.379, 55.1364) (-7.2357, 55.344) knots 0 0 0 1 2 2 2
  spline S73 degree 2 poles (-7.2357, 55.344) (-7.0923, 55.5467) (-6.64, 55.7444) (-6.3286, 55.7444) knots 0 0 0 1 2 2 2
  spline S74 degree 2 poles (-6.3286, 55.7444) (-5.9998, 55.7444) (-5.5599, 55.5368) (-5.419, 55.3316) knots 0 0 0 1 2 2 2
  spline S75 degree 2 poles (-5.419, 55.3316) (-5.2806, 55.1314) (-5.1545, 54.5407) (-5.1545, 54.1576) knots 0 0 0 1 2 2 2
  spline S76 degree 2 poles (-5.9232, 54.1576) (-5.9232, 54.7236) (-6.1086, 55.1809) (-6.3286, 55.1809) knots 0 0 0 1 2 2 2
  spline S77 degree 2 poles (-6.3286, 55.1809) (-6.5485, 55.1809) (-6.7364, 54.7236) (-6.7364, 54.1551) knots 0 0 0 1 2 2 2
  spline S78 degree 2 poles (-6.7364, 54.1551) (-6.7364, 53.5965) (-6.5485, 53.1319) (-6.3286, 53.1319) knots 0 0 0 1 2 2 2
  spline S79 degree 2 poles (-6.3286, 53.1319) (-6.1111, 53.1319) (-5.9232, 53.5965) (-5.9232, 54.1576) knots 0 0 0 1 2 2 2
  line L100 (-2.4432, 52.6326) -> (-4.6849, 52.6326)
  line L101 (-4.6849, 52.6326) -> (-4.6849, 53.1294)
  spline S80 degree 2 poles (-4.6849, 53.1294) (-4.4007, 53.3568) (-3.9459, 53.7572) (-3.7754, 53.9376) knots 0 0 0 1 2 2 2
  spline S81 degree 2 poles (-3.7754, 53.9376) (-3.5504, 54.1724) (-3.3502, 54.5308) (-3.3502, 54.7187) knots 0 0 0 1 2 2 2
  spline S82 degree 2 poles (-3.3502, 54.7187) (-3.3502, 54.9312) (-3.6048, 55.1586) (-3.8322, 55.1586) knots 0 0 0 1 2 2 2
  spline S83 degree 2 poles (-3.8322, 55.1586) (-3.9484, 55.1586) (-4.156, 55.1018) (-4.2623, 55.0573) knots 0 0 0 1 2 2 2
  spline S84 degree 2 poles (-4.2623, 55.0573) (-4.3661, 55.0103) (-4.5144, 54.9114) (-4.5515, 54.8867) knots 0 0 0 1 2 2 2
  line L102 (-4.5515, 54.8867) -> (-4.6108, 54.8867)
  line L103 (-4.6108, 54.8867) -> (-4.6108, 55.5516)
  spline S85 degree 2 poles (-4.6108, 55.5516) (-4.4823, 55.6134) (-3.9336, 55.7419) (-3.679, 55.7419) knots 0 0 0 1 2 2 2
  spline S86 degree 2 poles (-3.679, 55.7419) (-3.1352, 55.7419) (-2.5766, 55.2575) (-2.5766, 54.82) knots 0 0 0 1 2 2 2
  spline S87 degree 2 poles (-2.5766, 54.82) (-2.5766, 54.5506) (-2.8312, 54.0315) (-3.1253, 53.7349) knots 0 0 0 1 2 2 2
  spline S88 degree 2 poles (-3.1253, 53.7349) (-3.3107, 53.552) (-3.6592, 53.2678) (-3.7358, 53.2085) knots 0 0 0 1 2 2 2
  line L104 (-3.7358, 53.2085) -> (-2.4432, 53.2085)
  line L105 (-2.4432, 53.2085) -> (-2.4432, 52.6326)
  spline S89 degree 2 poles (0.2114, 53.6707) (0.2114, 53.1887) (-0.3991, 52.5683) (-0.933, 52.5683) knots 0 0 0 1 2 2 2
  spline S90 degree 2 poles (-0.933, 52.5683) (-1.1999, 52.5683) (-1.6176, 52.7216) (-1.7635, 52.8723) knots 0 0 0 1 2 2 2
  spline S91 degree 2 poles (-1.7635, 52.8723) (-1.9365, 53.0478) (-2.1218, 53.604) (-2.1218, 53.992) knots 0 0 0 1 2 2 2
  spline S92 degree 2 poles (-2.1218, 53.992) (-2.1218, 54.3924) (-1.9488, 55.0153) (-1.7536, 55.255) knots 0 0 0 1 2 2 2
  spline S93 degree 2 poles (-1.7536, 55.255) (-1.5682, 55.4824) (-0.9651, 55.7394) (-0.5524, 55.7394) knots 0 0 0 1 2 2 2
  spline S94 degree 2 poles (-0.5524, 55.7394) (-0.4016, 55.7394) (-0.1, 55.6999) (-0.0457, 55.6875) knots 0 0 0 1 2 2 2
  line L106 (-0.0457, 55.6875) -> (-0.0457, 55.0894)
  line L107 (-0.0457, 55.0894) -> (-0.1, 55.0894)
  spline S95 degree 2 poles (-0.1, 55.0894) (-0.1544, 55.1166) (-0.4016, 55.1833) (-0.5598, 55.1833) knots 0 0 0 1 2 2 2
  spline S96 degree 2 poles (-0.5598, 55.1833) (-0.9182, 55.1833) (-1.3087, 54.8052) (-1.3556, 54.4542) knots 0 0 0 1 2 2 2
  spline S97 degree 2 poles (-1.3556, 54.4542) (-1.2049, 54.5506) (-0.8959, 54.6643) (-0.7007, 54.6643) knots 0 0 0 1 2 2 2
  spline S98 degree 2 poles (-0.7007, 54.6643) (-0.5351, 54.6643) (-0.2459, 54.5753) (-0.1346, 54.4913) knots 0 0 0 1 2 2 2
  spline S99 degree 2 poles (-0.1346, 54.4913) (0.0235, 54.3702) (0.2114, 53.9772) (0.2114, 53.6707) knots 0 0 0 1 2 2 2
  spline S100 degree 2 poles (-0.6809, 53.211) (-0.6216, 53.2851) (-0.5573, 53.4581) (-0.5573, 53.6336) knots 0 0 0 1 2 2 2
  spline S101 degree 2 poles (-0.5573, 53.6336) (-0.5573, 53.7819) (-0.6314, 53.9747) (-0.6982, 54.0315) knots 0 0 0 1 2 2 2
  spline S102 degree 2 poles (-0.6982, 54.0315) (-0.7674, 54.0909) (-0.9379, 54.1329) (-1.0343, 54.1329) knots 0 0 0 1 2 2 2
  spline S103 degree 2 poles (-1.0343, 54.1329) (-1.1159, 54.1329) (-1.284, 54.0909) (-1.3581, 54.0612) knots 0 0 0 1 2 2 2
  spline S104 degree 2 poles (-1.3581, 54.0612) (-1.3581, 54.0414) (-1.3631, 53.9475) (-1.3631, 53.8758) knots 0 0 0 1 2 2 2
  spline S105 degree 2 poles (-1.3631, 53.8758) (-1.3631, 53.6114) (-1.2716, 53.2925) (-1.1999, 53.211) knots 0 0 0 1 2 2 2
  spline S106 degree 2 poles (-1.1999, 53.211) (-1.148, 53.1442) (-1.0096, 53.0874) (-0.9355, 53.0874) knots 0 0 0 1 2 2 2
  spline S107 degree 2 poles (-0.9355, 53.0874) (-0.8737, 53.0874) (-0.7303, 53.1492) (-0.6809, 53.211) knots 0 0 0 1 2 2 2
  point P0 (0, 0)
  dimension "d4" = 19
  constraints: 2 other
extrude "Extrusion35" add sketch "Sketch39" along normal blind 2
sketch "Sketch40" plane through (0, 15, 0) normal (0, 1, 0) x (1, 0, 0)
  line L0 (55.24, 30) -> (64.95, 30) construction
  line L1 (64.95, 30) -> (64.95, 57.7) construction
  line L2 (64.95, 57.7) -> (29.25, 57.7) construction
  line L3 (29.25, 57.7) -> (29.25, 62.7) construction
  line L4 (-52.75, 62.7) -> (29.25, 62.7) construction
  line L5 (-52.75, 57.7) -> (-52.75, 62.7) construction
  line L6 (-52.75, 57.7) -> (-88.45, 57.7) construction
  line L7 (-88.45, 57.7) -> (-88.45, 30) construction
  line L8 (-88.45, 30) -> (-78.7093, 30) construction
  arc A0 (-75.7093, 27) -> (-78.7093, 30) centre (-78.7093, 27) ccw construction
  line L9 (-75.7093, 27) -> (-75.7093, -27) construction
  arc A1 (-78.7093, -30) -> (-75.7093, -27) centre (-78.7093, -27) ccw construction
  line L10 (-78.7093, -30) -> (-88.45, -30) construction
  line L11 (-88.45, -30) -> (-88.45, -57.7) construction
  line L12 (-88.45, -57.7) -> (-52.75, -57.7) construction
  line L13 (-52.75, -62.4308) -> (-52.75, -57.7) construction
  line L14 (29.25, -62.4308) -> (-52.75, -62.4308) construction
  line L15 (29.25, -62.4308) -> (29.25, -57.7) construction
  line L16 (29.25, -57.7) -> (64.95, -57.7) construction
  line L17 (64.95, -57.7) -> (64.95, -30) construction
  line L18 (64.95, -30) -> (55.24, -30) construction
  arc A2 (52.24, -27) -> (55.24, -30) centre (55.24, -27) ccw construction
  line L19 (52.24, -27) -> (52.24, 27) construction
  arc A3 (55.24, 30) -> (52.24, 27) centre (55.24, 27) ccw construction
  line L20 (36.5, 5) -> (36.5, -5) construction
  arc A4 (34.5, -5) -> (36.5, -5) centre (35.5, -5) ccw construction
  line L21 (34.5, -5) -> (34.5, 5) construction
  arc A5 (36.5, 5) -> (34.5, 5) centre (35.5, 5) ccw construction
  line L22 (49.7398, 0) -> (46.6799, -5.3) construction
  line L23 (46.6799, -5.3) -> (40.56, -5.3) construction
  line L24 (40.56, -5.3) -> (37.5, 0) construction
  line L25 (37.5, 0) -> (40.56, 5.3) construction
  line L26 (40.56, 5.3) -> (46.6799, 5.3) construction
  line L27 (46.6799, 5.3) -> (49.7398, 0) construction
  line L28 (-58, 5) -> (-58, -5) construction
  arc A6 (-60, -5) -> (-58, -5) centre (-59, -5) ccw construction
  line L29 (-60, -5) -> (-60, 5) construction
  arc A7 (-58, 5) -> (-60, 5) centre (-59, 5) ccw construction
  line L30 (-70.1799, -5.3) -> (-73.2398, 0) construction
  line L31 (-73.2398, 0) -> (-70.1799, 5.3) construction
  line L32 (-70.1799, 5.3) -> (-64.06, 5.3) construction
  line L33 (-64.06, 5.3) -> (-61, 0) construction
  line L34 (-61, 0) -> (-64.06, -5.3) construction
  line L35 (-64.06, -5.3) -> (-70.1799, -5.3) construction
  circle A8 centre (23.5, 0) radius 9.5 construction
  circle A9 centre (-35.25, 20.3516) radius 9.5 construction
  circle A10 centre (-11.75, 20.3516) radius 9.5 construction
  circle A11 centre (11.75, 20.3516) radius 9.5 construction
  circle A12 centre (-35.25, -20.3516) radius 9.5 construction
  circle A13 centre (-11.75, -20.3516) radius 9.5 construction
  circle A14 centre (11.75, -20.3516) radius 9.5 construction
  circle A15 centre (-23.5, 0) radius 9.5 construction
  circle A16 centre (0, 0) radius 9.5 construction
  circle A17 centre (-47, 0) radius 9.5 construction
  circle A18 centre (-23.5, 43.85) radius 3.5
  circle A19 centre (0, 43.85) radius 3.5
  circle A20 centre (-23.5, -43.85) radius 3.5
  circle A21 centre (0, -43.85) radius 3.5
  dimension "d367" = 7
  dimension "d368" = 7
  dimension "d369" = 7
  dimension "d370" = 7
  constraints: 4 centre point
  measures "d367" diameter of A18
  measures "d368" diameter of A19
  measures "d369" diameter of A20
  measures "d370" diameter of A21
extrude "Extrusion36" cut sketch "Sketch40" against normal through all
body "Solid1"
